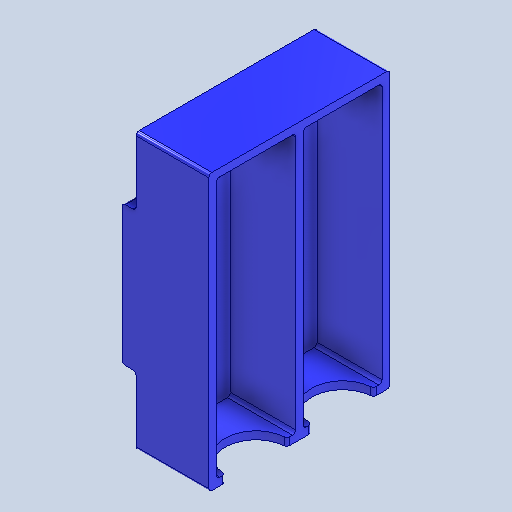
# Autodesk Inventor part: roja-v1-3DP-lipo-box
Saved by Autodesk Inventor 2025.2 (Build 292293000, 293)
## iProperties
Created: 2024-08-20
Part Number: roja-v1-3DP-lipo-box
Material: ABS プラスチック
Document SubType Name: Modeling
Designer: haruy
Density: 1.06 g/cm^3
Appearance: 青 - 壁塗料 - 光沢
Author: haruy
Autodesk Inventor part; units mm, degrees
ref_plane "YZ Plane" through (0, 0, 0) normal (1, 0, 0) x (0, 1, 0)
ref_plane "XZ Plane" through (0, 0, 0) normal (0, 1, 0) x (-1, 0, 0)
ref_plane "XY Plane" through (0, 0, 0) normal (0, 0, 1) x (1, 0, 0)
sketch "スケッチ1" plane through (0, 0, 0) normal (1, 0, 0) x (0, 1, 0)
  line L0 (0, 0) -> (155, 0)
  line L1 (155, 0) -> (155, -45)
  line L2 (155, -45) -> (0, -45)
  line L3 (0, -45) -> (0, 0)
  line L4 (155, -56) -> (0, -56)
  line L5 (0, -56) -> (0, -101)
  line L6 (0, -101) -> (155, -101)
  line L7 (155, -101) -> (155, -56)
  line L8 (158, 3) -> (-20, 3)
  line L9 (-20, 3) -> (-20, -104)
  line L10 (-20, -104) -> (158, -104)
  line L11 (158, -104) -> (158, 3)
  line L12 (-20, 36.5) -> (-40, 36.5)
  line L13 (-40, 36.5) -> (-40, -137.5)
  line L14 (-40, -137.5) -> (-20, -137.5)
  line L15 (-20, -137.5) -> (-20, 36.5)
  line L16 (163, 8) -> (-25, 8)
  line L17 (-25, 8) -> (-25, -109)
  line L18 (-25, -109) -> (163, -109)
  line L19 (163, -109) -> (163, 8)
  line L20 (-20, 8) -> (-15, 8)
  line L21 (-15, 8) -> (-15, 28)
  line L22 (-15, 28) -> (-20, 28)
  line L23 (-20, 28) -> (-20, 8)
  line L24 (-15, 18) -> (-20, 18)
  line L25 (158, -48) -> (-20, -48)
  line L26 (-20, -48) -> (-20, -53)
  line L27 (-20, -53) -> (158, -53)
  line L28 (158, -53) -> (158, -48)
  line L29 (-20, -109) -> (-15, -109)
  line L30 (-15, -109) -> (-15, -129)
  line L31 (-15, -129) -> (-20, -129)
  line L32 (-20, -129) -> (-20, -109)
  line L33 (-15, -109) -> (-10, -109)
  line L34 (-10, -109) -> (-10, 8)
  line L35 (-10, 8) -> (-15, 8)
  line L36 (-15, 8) -> (-15, -109)
  line L37 (64, 8) -> (84, 8)
  line L38 (84, 8) -> (84, 13)
  line L39 (84, 13) -> (64, 13)
  line L40 (64, 13) -> (64, 8)
  line L41 (74, 13) -> (74, 8)
  line L42 (158, -50.5) -> (-10, -50.5)
  line L43 (64, -109) -> (84, -109)
  line L44 (84, -109) -> (84, -114)
  line L45 (84, -114) -> (64, -114)
  line L46 (64, -114) -> (64, -109)
  line L47 (74, -114) -> (74, -109)
  point P0 (-20, 3)
  point P1 (158, -53)
  point P2 (74, 10.5)
  point P3 (74, -111.5)
  point P4 (-10, 3)
  point P5 (-10, -48)
  point P6 (-10, -53)
  point P7 (-10, -104)
  point P8 (-10, 8)
  dimension "d2" = 155
  dimension "d3" = 45
  dimension "d4" = 155
  dimension "d5" = 45
  dimension "d6" = 11
  dimension "d7" = 0
  dimension "d8" = 3
  dimension "d9" = 3
  dimension "d10" = 3
  dimension "d11" = 20
  dimension "d12" = 20
  dimension "d13" = 174
  dimension "d15" = 33.5
  dimension "d16" = 0
  dimension "d17" = 5
  dimension "d18" = 5
  dimension "d19" = 20
  dimension "d20" = 5
  dimension "d21" = 3
  dimension "d22" = 5
  dimension "d23" = 20
  dimension "d42" = 5
  dimension "d43" = 0
  dimension "d44" = 10
  dimension "d45" = 20
  dimension "d46" = 5
  dimension "d47" = 89
  constraints: 96 end point, 20 parallel, 10 perpendicular, 9 horizontal, 8 point on line, 7 midpoint, 7 symmetric about line, 3 other
  measures "d2" distance of L1.end L2.end
  measures "d3" distance of L0.end L1.end
  measures "d4" distance of L6.end L5.end
  measures "d5" distance of L5.end L4.end
  measures "d6" distance between parallel lines of L2 L4
  measures "d7" distance between parallel lines of L3 L5
  measures "d8" distance between parallel lines of L8 L0
  measures "d9" distance between parallel lines of L6 L10
  measures "d10" distance between parallel lines of L7 L11
  measures "d11" distance between parallel lines of L3 L9
  measures "d12" distance of L14.end L13.end
  measures "d13" distance of L12.end L13.end
  measures "d15" distance between parallel lines of L12 L8
  measures "d16" distance between parallel lines of L9 L15
  measures "d17" distance between parallel lines of L11 L19
  measures "d18" distance of L22.end L21.end
  measures "d19" distance of L21.end L20.end
  measures "d20" distance between parallel lines of L27 L25
  measures "d21" distance between parallel lines of L2 L25
  measures "d22" distance of L30.end L31.end
  measures "d23" distance of L29.end L30.end
  measures "d42" distance of L35.end L34.end
  measures "d43" distance between parallel lines of L35 L16
  measures "d44" distance between parallel lines of L34 L3
  measures "d45" distance of L39.end L38.end
  measures "d46" distance of L38.end L37.end
  measures "d47" distance from line of L19 point (74, 10.5)
extrude "押し出し1" add sketch "スケッチ1" along normal blind 47 contours L8 L34 L16 L19 L18 L10 L11 | L34 L25 L36 L8 | L8 L36 L16 L34 | L11 L42 L34 L25 | L34 L27 L36 L25 | L11 L27 L34 L42 | L27 L34 L10 L36 | L10 L34 L18 L36
extrude "押し出し3" add sketch "スケッチ1" along normal blind 5 contours L0 L1 L2 L3 | L7 L6 L5 L4 | L11 L25 L34 L8 | L8 L34 L16 L19 L18 L10 L11 | L11 L10 L34 L27
sketch "スケッチ3" plane through (47, -15, -109) normal (0, 0, -1) x (-1, 0, 0)
  point P0 (47, 15)
sketch "スケッチ4" plane through (0, -15, -109) normal (0, 0, -1) x (-1, 0, 0)
  line L0 (0, 0) -> (-47, 0) projected
  line L1 (0, 178) -> (-47, 178) projected
  line L2 (-32, 0) -> (-20, 0)
  line L3 (-20, 0) -> (-20, 178)
  line L4 (-20, 178) -> (-32, 178)
  line L5 (-32, 178) -> (-32, 0)
  line L6 (0, 0) -> (0, 178) projected
  line L7 (-20, 84) -> (-32, 84)
  line L8 (-32, 84) -> (-32, 104)
  line L9 (-32, 104) -> (-20, 104)
  line L10 (-20, 104) -> (-20, 84)
  line L11 (-32, 94) -> (-20, 94)
  circle A0 centre (-26, 94) radius 3.5
  circle A1 centre (-26, 84) radius 3.5
  line L12 (-20, 84) -> (-32, 84)
  line L13 (-32, 84) -> (-32, 74)
  line L14 (-32, 74) -> (-20, 74)
  line L15 (-20, 74) -> (-20, 84)
  point P0 (0, 15)
  point P1 (-32, 84)
  point P2 (-20, 104)
  point P3 (-32, 104)
  point P4 (-32, 74)
  point P5 (-20, 74)
  dimension "d48" = 12
  dimension "d49" = 20
  dimension "d50" = 12
  dimension "d51" = 20
  dimension "d52" = 84
  dimension "d69" = 7
  dimension "d80" = 10
  dimension "d81" = 6
  dimension "d82" = 7
  dimension "d83" = 12
  dimension "d84" = 10
  constraints: 26 end point, 6 parallel, 3 horizontal, 3 midpoint, 3 perpendicular, 3 point on line, 2 centre point, 2 coincident
  measures "d48" distance of L4.end L3.end
  measures "d49" distance between parallel lines of L6 L3
  measures "d50" distance of L8.end L9.end
  measures "d51" distance of L7.end L8.end
  measures "d52" distance between parallel lines of L1 L11
  measures "d69" diameter of A0
  measures "d80" distance of A0.centre point (-26, 84)
  measures "d81" distance from line of L5 point (-26, 84)
  measures "d82" diameter of A1
  measures "d83" distance of L14.end L13.end
  measures "d84" distance of L13.end L12.end
sketch "スケッチ5" plane through (0, -15, -109) normal (0, -1, 0) x (1, 0, 0)
  line L0 (47, 117) -> (47, 0) projected
  circle A0 centre (47, 86.5) radius 20
  line L1 (0, 117) -> (47, 117) projected
  circle A1 centre (47, 30.5) radius 20
  line L2 (0, 0) -> (47, 0) projected
  point P0 (0, 109)
  point P1 (47, 10.5)
  point P2 (47, 50.5)
  point P3 (47, 66.5)
  point P4 (47, 106.5)
  dimension "d72" = 40
  dimension "d73" = 30.5
  dimension "d74" = 40
  dimension "d75" = 30.5
  constraints: 2 centre point, 2 point on line
  measures "d72" diameter of A0
  measures "d73" distance from line of A0.centre L1
  measures "d74" diameter of A1
  measures "d75" distance from line of L2 A1.centre
extrude "押し出し6" cut sketch "スケッチ5" against normal blind 18.875 contours L0 A0 | L0 A1 picked at (42.3064, 80.4032) picked at (35.4972, 35.77)
ref_plane "作業平面1" through (47, -10, -50.5) normal (0, 0, -1) x (-1, 0, 0)
fillet "フィレット2" radius 2 16 edges at (23.5, 163, 8) (23.5, 163, -109) (23.5, -15, -109) (23.5, -15, 8) (47, -12.5, -2.5) (47, -12.5, -42.5) (47, -12.5, -58.5) (47, -12.5, -98.5) (26, -10, -53) (26, -10, -104) (26, 158, -53) (26, 158, -104) (26, -10, 3) (26, -10, -48) (26, 158, -48) (26, 158, 3)
sketch "スケッチ6" plane through (0, 0, 0) normal (-1, 0, 0) x (0, 0, 1)
  line L0 (8, 161) -> (8, -13) projected
  line L1 (8, 119) -> (-152.9201, 119)
  line L2 (-152.9201, 119) -> (-152.9201, 99)
  line L3 (-152.9201, 99) -> (8, 99)
  line L4 (8, 99) -> (8, 119)
  line L5 (8, 49) -> (-150.1985, 49)
  line L6 (-150.1985, 49) -> (-150.1985, 29)
  line L7 (-150.1985, 29) -> (8, 29)
  line L8 (8, 29) -> (8, 49)
  line L9 (-107, 163) -> (6, 163) projected
  line L10 (-72, 119) -> (-72, 29)
  circle A0 centre (-21, 109) radius 1.7
  circle A1 centre (-61.5, 109) radius 1.7
  line L11 (8, 74) -> (-109, 74)
  line L12 (-109, -13) -> (-109, 161) projected
  circle A2 centre (-21, 39) radius 1.7
  circle A3 centre (-61.5, 39) radius 1.7
  line L13 (-71, 119) -> (-71, 29)
  line L14 (8, 119) -> (8, 29)
  point P0 (0, 0)
  dimension "d85" = 20
  dimension "d86" = 20
  dimension "d87" = 50
  dimension "d88" = 44
  dimension "d89" = 80
  dimension "d90" = 3.4
  dimension "d91" = 3.4
  dimension "d92" = 29
  dimension "d93" = 10
  dimension "d94" = 40.5
  dimension "d95" = 10
  dimension "d96" = 1
  constraints: 24 end point, 6 point on line, 4 centre point, 4 parallel, 4 perpendicular, 2 horizontal, 2 midpoint, 2 symmetric about line, 1 vertical, 2 other
  measures "d85" distance of L2.end L1.end
  measures "d86" distance of L6.end L5.end
  measures "d87" distance between parallel lines of L3 L5
  measures "d88" distance between parallel lines of L9 L1
  measures "d89" distance between parallel lines of L10 L0
  measures "d90" diameter of A0
  measures "d91" diameter of A1
  measures "d92" distance from line of A0.centre L4
  measures "d93" distance from line of A0.centre L3
  measures "d94" distance of A0.centre A1.centre
  measures "d95" distance from line of L3 A1.centre
  measures "d96" distance between parallel lines of L10 L13
extrude "押し出し7" add sketch "スケッチ6" along normal blind 9 contours L0 L3 L13 L1 | L0 L11 L13 L3 | L0 L5 L13 L11 | L0 L7 L13 L5
hole "穴4" at (0, 109, -21) at (0, 109, -61.5) at (0, 39, -61.5) at (0, 39, -21) direction (1, 0, 0) diameter 3.4 end through all
sketch "スケッチ7" plane through (5, 0, 0) normal (1, 0, 0) x (0, 0, -1)
  circle A0 centre (21, 109) radius 1.7 projected
  circle A1 centre (21, 109) radius 4
  circle A2 centre (61.5, 109) radius 1.7 projected
  circle A3 centre (61.5, 109) radius 4
  circle A4 centre (21, 39) radius 1.7 projected
  circle A5 centre (21, 39) radius 4
  circle A6 centre (61.5, 39) radius 1.7 projected
  circle A7 centre (61.5, 39) radius 4
  point P0 (0, 0)
  dimension "d106" = 8
  dimension "d107" = 8
  dimension "d108" = 8
  dimension "d109" = 8
  constraints: 4 centre point, 4 coincident
  measures "d106" diameter of A1
  measures "d107" diameter of A3
  measures "d108" diameter of A5
  measures "d109" diameter of A7
extrude "押し出し8" cut sketch "スケッチ7" against normal blind 3 contours A0 | A1 | A2 | A3 | A4 | A5 | A6 | A7
fillet "フィレット3" radius 2 6 edges at (0, 29, -31.5) (-9, 29, -31.5) (0, 74, -71) (-9, 74, -71) (0, 119, -31.5) (-9, 119, -31.5)
equation "\"d95\" = d93"
